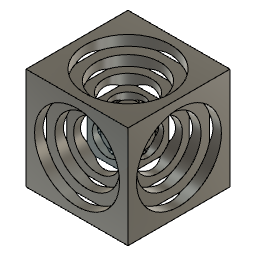
turnerscube (Autodesk Fusion 360 design; units mm, degrees)
Autodesk Fusion 360 part; units mm, degrees
note: some values were not read from the file. Set by a fixed rule: which sketch regions a step uses.
sketch "Sketch1" plane through (0, 0, 0) normal (0, 0, 1) x (1, 0, 0)
  line L0 (0, 0) -> (30, 0)
  line L1 (30, 0) -> (30, 30)
  line L2 (30, 30) -> (0, 30)
  line L3 (0, 30) -> (0, 0)
  dimension "d1" = 30
  dimension "d2" = 30
  constraint horizontal L0
  constraint vertical L1
  constraint horizontal L2
  constraint vertical L3
  constraint coincident L0.start L3.end
  measures "d1" distance of L0.start L2.end
  measures "d2" distance of L0.start L0.end
extrude "Extrude1" add sketch "Sketch1" along normal blind 30
sketch "Sketch2" plane through (30, 0, 0) normal (1, 0, 0) x (0, 1, 0)
  line L0 (0, 0) -> (30, 0)
  line L1 (30, 0) -> (30, 30)
  line L2 (30, 30) -> (0, 30)
  line L3 (0, 30) -> (0, 0)
  circle A0 centre (15, 15) radius 12.5
  line L4 (15, 30) -> (15, 0)
  dimension "d5" = 25
  constraint midpoint L2 L4.start
  constraint midpoint L0 L4.end
  constraint coincident A0.centre L4
  constraint midpoint A0.centre L4
  measures "d5" diameter of A0
  measures "d43" diameter of L2.end
sketch "Sketch3" plane through (0, 0, 30) normal (0, 0, 1) x (-1, 0, 0)
  line L0 (0, -30) -> (0, 0)
  line L1 (0, 0) -> (-30, 0)
  line L2 (-30, 0) -> (-30, -30)
  line L3 (-30, -30) -> (0, -30)
  circle A0 centre (-15, -15) radius 12.5
  line L4 (-15, -30) -> (-15, 0)
  dimension "d6" = 25
  constraint midpoint L3 L4.start
  constraint midpoint L1 L4.end
  constraint midpoint A0.centre L4
  measures "d6" diameter of A0
sketch "Sketch4" plane through (0, 0, 0) normal (0, -1, 0) x (1, 0, 0)
  line L0 (0, 0) -> (30, 0)
  line L1 (30, 0) -> (30, 30)
  line L2 (30, 30) -> (0, 30)
  line L3 (0, 30) -> (0, 0)
  circle A0 centre (15, 15) radius 12.5
  line L4 (15, 30) -> (15, 0)
  dimension "d7" = 25
  constraint midpoint L2 L4.start
  constraint midpoint L0 L4.end
  constraint midpoint A0.centre L4
  measures "d7" diameter of A0
sketch "Sketch5" plane through (0, 30, 0) normal (0, 1, 0) x (-1, 0, 0)
  line L0 (-30, 0) -> (0, 0)
  line L1 (0, 0) -> (0, 30)
  line L2 (0, 30) -> (-30, 30)
  line L3 (-30, 30) -> (-30, 0)
  circle A0 centre (-15, 15) radius 12.5
  line L4 (-15, 30) -> (-15, 0)
  dimension "d8" = 25
  constraint midpoint L2 L4.start
  constraint midpoint L0 L4.end
  constraint midpoint A0.centre L4
  measures "d8" diameter of A0
sketch "Sketch6" plane through (0, 0, 0) normal (-1, 0, 0) x (0, -1, 0)
  line L0 (-30, 0) -> (0, 0)
  line L1 (0, 0) -> (0, 30)
  line L2 (0, 30) -> (-30, 30)
  line L3 (-30, 30) -> (-30, 0)
  line L4 (-15, 30) -> (-15, 0)
  circle A0 centre (-15, 15) radius 12.5
  dimension "d9" = 25
  constraint midpoint L2 L4.start
  constraint midpoint L0 L4.end
  constraint midpoint L4 A0.centre
  measures "d9" diameter of A0
sketch "Sketch7" plane through (0, 0, 0) normal (0, 0, -1) x (1, 0, 0)
  line L0 (0, 0) -> (0, -30)
  line L1 (0, -30) -> (30, -30)
  line L2 (30, -30) -> (30, 0)
  line L3 (30, 0) -> (0, 0)
  line L4 (15, 0) -> (15, -30)
  circle A0 centre (15, -15) radius 12.5
  dimension "d10" = 25
  constraint midpoint L3 L4.start
  constraint midpoint L1 L4.end
  constraint midpoint L4 A0.centre
  measures "d10" diameter of A0
extrude "Extrude2" cut sketch "Sketch2" against normal blind 3 contours A0 L4 | A0 L4
extrude "Extrude3" cut sketch "Sketch4" against normal blind 3 contours A0 L4 | A0 L4
extrude "Extrude4" cut sketch "Sketch3" against normal blind 3 contours A0 L4 | A0 L4
extrude "Extrude5" cut sketch "Sketch5" against normal blind 3 contours A0 L4 | A0 L4
extrude "Extrude6" cut sketch "Sketch7" against normal blind 3 contours L4 A0 | L4 A0
extrude "Extrude7" cut sketch "Sketch6" against normal blind 3 contours L4 A0 | L4 A0
sketch "Sketch8" plane through (27, 0, 0) normal (1, 0, 0) x (0, 1, 0)
  line L0 (11.5, 3) -> (18.5, 3)
  arc A0 (18.5, 3) -> (27, 11.5) centre (15, 15) ccw
  line L1 (27, 11.5) -> (27, 18.5)
  arc A1 (27, 18.5) -> (18.5, 27) centre (15, 15) ccw
  line L2 (18.5, 27) -> (11.5, 27)
  arc A2 (11.5, 27) -> (3, 18.5) centre (15, 15) ccw
  line L3 (3, 18.5) -> (3, 11.5)
  arc A3 (3, 11.5) -> (11.5, 3) centre (15, 15) ccw
  circle A4 centre (15, 15) radius 9.5
  line L4 (15, 27) -> (15, 3)
  dimension "d23" = 19
  constraint midpoint L2 L4.start
  constraint midpoint L0 L4.end
  constraint midpoint A0.centre L4
  measures "d23" diameter of A4
sketch "Sketch9" plane through (0, 0, 27) normal (0, 0, 1) x (-1, 0, 0)
  line L0 (-3, -18.5) -> (-3, -11.5)
  arc A0 (-3, -11.5) -> (-11.5, -3) centre (-15, -15) ccw
  line L1 (-11.5, -3) -> (-18.5, -3)
  arc A1 (-18.5, -3) -> (-27, -11.5) centre (-15, -15) ccw
  line L2 (-27, -11.5) -> (-27, -18.5)
  arc A2 (-27, -18.5) -> (-18.5, -27) centre (-15, -15) ccw
  line L3 (-18.5, -27) -> (-11.5, -27)
  arc A3 (-11.5, -27) -> (-3, -18.5) centre (-15, -15) ccw
  line L4 (-15, -27) -> (-15, -3)
  circle A4 centre (-15, -15) radius 9.5
  dimension "d24" = 19
  constraint midpoint L3 L4.start
  constraint midpoint L1 L4.end
  constraint midpoint L4 A0.centre
  measures "d24" diameter of A4
sketch "Sketch10" plane through (0, 3, 0) normal (0, -1, 0) x (1, 0, 0)
  line L0 (3, 18.5) -> (3, 11.5)
  arc A0 (3, 11.5) -> (11.5, 3) centre (15, 15) ccw
  line L1 (11.5, 3) -> (18.5, 3)
  arc A1 (18.5, 3) -> (27, 11.5) centre (15, 15) ccw
  line L2 (27, 11.5) -> (27, 18.5)
  arc A2 (27, 18.5) -> (18.5, 27) centre (15, 15) ccw
  line L3 (18.5, 27) -> (11.5, 27)
  arc A3 (11.5, 27) -> (3, 18.5) centre (15, 15) ccw
  line L4 (15, 27) -> (15, 3)
  circle A4 centre (15, 15) radius 9.5
  dimension "d25" = 19
  constraint midpoint L3 L4.start
  constraint midpoint L1 L4.end
  constraint midpoint L4 A0.centre
  measures "d25" diameter of A4
sketch "Sketch11" plane through (3, 0, 0) normal (-1, 0, 0) x (0, -1, 0)
  line L0 (-18.5, 3) -> (-11.5, 3)
  arc A0 (-11.5, 3) -> (-3, 11.5) centre (-15, 15) ccw
  line L1 (-3, 11.5) -> (-3, 18.5)
  arc A1 (-3, 18.5) -> (-11.5, 27) centre (-15, 15) ccw
  line L2 (-11.5, 27) -> (-18.5, 27)
  arc A2 (-18.5, 27) -> (-27, 18.5) centre (-15, 15) ccw
  line L3 (-27, 18.5) -> (-27, 11.5)
  arc A3 (-27, 11.5) -> (-18.5, 3) centre (-15, 15) ccw
  line L4 (-15, 27) -> (-15, 3)
  circle A4 centre (-15, 15) radius 9.5
  dimension "d26" = 19
  constraint midpoint L2 L4.start
  constraint midpoint L0 L4.end
  constraint midpoint L4 A0.centre
  measures "d26" diameter of A4
sketch "Sketch12" plane through (0, 27, 0) normal (0, 1, 0) x (-1, 0, 0)
  line L0 (-3, 11.5) -> (-3, 18.5)
  arc A0 (-3, 18.5) -> (-11.5, 27) centre (-15, 15) ccw
  line L1 (-11.5, 27) -> (-18.5, 27)
  arc A1 (-18.5, 27) -> (-27, 18.5) centre (-15, 15) ccw
  line L2 (-27, 18.5) -> (-27, 11.5)
  arc A2 (-27, 11.5) -> (-18.5, 3) centre (-15, 15) ccw
  line L3 (-18.5, 3) -> (-11.5, 3)
  arc A3 (-11.5, 3) -> (-3, 11.5) centre (-15, 15) ccw
  line L4 (-15, 27) -> (-15, 3)
  circle A4 centre (-15, 15) radius 9.5
  dimension "d27" = 19
  constraint midpoint L1 L4.start
  constraint midpoint L3 L4.end
  constraint concentric A0 A4
  measures "d27" diameter of A4
sketch "Sketch13" plane through (0, 0, 3) normal (0, 0, -1) x (1, 0, 0)
  line L0 (3, -11.5) -> (3, -18.5)
  arc A0 (3, -18.5) -> (11.5, -27) centre (15, -15) ccw
  line L1 (11.5, -27) -> (18.5, -27)
  arc A1 (18.5, -27) -> (27, -18.5) centre (15, -15) ccw
  line L2 (27, -18.5) -> (27, -11.5)
  arc A2 (27, -11.5) -> (18.5, -3) centre (15, -15) ccw
  line L3 (18.5, -3) -> (11.5, -3)
  arc A3 (11.5, -3) -> (3, -11.5) centre (15, -15) ccw
  line L4 (15, -3) -> (15, -27)
  circle A4 centre (15, -15) radius 9.5
  dimension "d28" = 19
  constraint midpoint L3 L4.start
  constraint midpoint L1 L4.end
  constraint concentric A0 A4
  measures "d28" diameter of A4
extrude "Extrude8" cut sketch "Sketch13" against normal blind 3 contours L4 A4 | L4 A4
extrude "Extrude9" cut sketch "Sketch12" against normal blind 3 contours L4 A4 | L4 A4
extrude "Extrude10" cut sketch "Sketch9" against normal blind 3 contours L4 A4 | L4 A4
extrude "Extrude11" cut sketch "Sketch8" against normal blind 3 contours A4 L4 | A4 L4
extrude "Extrude12" cut sketch "Sketch10" against normal blind 3 contours L4 A4 | L4 A4
extrude "Extrude13" cut sketch "Sketch11" against normal blind 3 contours L4 A4 | L4 A4
sketch "Sketch14" plane through (0, 24, 0) normal (0, 1, 0) x (-1, 0, 0)
  line L0 (-6, 11.9586) -> (-6, 18.0414)
  arc A0 (-6, 18.0414) -> (-11.9586, 24) centre (-15, 15) ccw
  line L1 (-11.9586, 24) -> (-18.0414, 24)
  arc A1 (-18.0414, 24) -> (-24, 18.0414) centre (-15, 15) ccw
  line L2 (-24, 18.0414) -> (-24, 11.9586)
  arc A2 (-24, 11.9586) -> (-18.0414, 6) centre (-15, 15) ccw
  line L3 (-18.0414, 6) -> (-11.9586, 6)
  arc A3 (-11.9586, 6) -> (-6, 11.9586) centre (-15, 15) ccw
  line L4 (-15, 24) -> (-15, 6)
  circle A4 centre (-15, 15) radius 7
  dimension "d41" = 14
  constraint midpoint L1 L4.start
  constraint midpoint L3 L4.end
  constraint concentric A0 A4
  measures "d41" diameter of A4
sketch "Sketch15" plane through (6, 0, 0) normal (-1, 0, 0) x (0, -1, 0)
  line L0 (-6, 11.9586) -> (-6, 18.0414)
  arc A0 (-6, 18.0414) -> (-11.9586, 24) centre (-15, 15) ccw
  line L1 (-11.9586, 24) -> (-18.0414, 24)
  arc A1 (-18.0414, 24) -> (-24, 18.0414) centre (-15, 15) ccw
  line L2 (-24, 18.0414) -> (-24, 11.9586)
  arc A2 (-24, 11.9586) -> (-18.0414, 6) centre (-15, 15) ccw
  line L3 (-18.0414, 6) -> (-11.9586, 6)
  arc A3 (-11.9586, 6) -> (-6, 11.9586) centre (-15, 15) ccw
  line L4 (-15, 24) -> (-15, 6)
  circle A4 centre (-15, 15) radius 7
  dimension "d42" = 14
  constraint midpoint L1 L4.start
  constraint midpoint L3 L4.end
  constraint concentric A0 A4
  measures "d42" diameter of A4
sketch "Sketch16" plane through (0, 6, 0) normal (0, -1, 0) x (1, 0, 0)
  line L0 (6, 18.0414) -> (6, 11.9586)
  arc A0 (6, 11.9586) -> (11.9586, 6) centre (15, 15) ccw
  line L1 (11.9586, 6) -> (18.0414, 6)
  arc A1 (18.0414, 6) -> (24, 11.9586) centre (15, 15) ccw
  line L2 (24, 11.9586) -> (24, 18.0414)
  arc A2 (24, 18.0414) -> (18.0414, 24) centre (15, 15) ccw
  line L3 (18.0414, 24) -> (11.9586, 24)
  arc A3 (11.9586, 24) -> (6, 18.0414) centre (15, 15) ccw
  line L4 (15, 24) -> (15, 6)
  circle A4 centre (15, 15) radius 7
  dimension "d43" = 14
  constraint midpoint L3 L4.start
  constraint midpoint L1 L4.end
  constraint concentric A0 A4
  measures "d43" diameter of A4
sketch "Sketch17" plane through (24, 0, 0) normal (1, 0, 0) x (0, 1, 0)
  line L0 (6, 18.0414) -> (6, 11.9586)
  arc A0 (6, 11.9586) -> (11.9586, 6) centre (15, 15) ccw
  line L1 (11.9586, 6) -> (18.0414, 6)
  arc A1 (18.0414, 6) -> (24, 11.9586) centre (15, 15) ccw
  line L2 (24, 11.9586) -> (24, 18.0414)
  arc A2 (24, 18.0414) -> (18.0414, 24) centre (15, 15) ccw
  line L3 (18.0414, 24) -> (11.9586, 24)
  arc A3 (11.9586, 24) -> (6, 18.0414) centre (15, 15) ccw
  line L4 (15, 24) -> (15, 6)
  circle A4 centre (15, 15) radius 7
  dimension "d44" = 14
  constraint midpoint L3 L4.start
  constraint midpoint L1 L4.end
  constraint concentric A0 A4
  measures "d44" diameter of A4
sketch "Sketch18" plane through (0, 0, 24) normal (0, 0, 1) x (-1, 0, 0)
  line L0 (-6, -18.0414) -> (-6, -11.9586)
  arc A0 (-6, -11.9586) -> (-11.9586, -6) centre (-15, -15) ccw
  line L1 (-11.9586, -6) -> (-18.0414, -6)
  arc A1 (-18.0414, -6) -> (-24, -11.9586) centre (-15, -15) ccw
  line L2 (-24, -11.9586) -> (-24, -18.0414)
  arc A2 (-24, -18.0414) -> (-18.0414, -24) centre (-15, -15) ccw
  line L3 (-18.0414, -24) -> (-11.9586, -24)
  arc A3 (-11.9586, -24) -> (-6, -18.0414) centre (-15, -15) ccw
  line L4 (-15, -24) -> (-15, -6)
  circle A4 centre (-15, -15) radius 7
  dimension "d45" = 14
  constraint midpoint L3 L4.start
  constraint midpoint L1 L4.end
  constraint concentric A0 A4
  measures "d45" diameter of A4
sketch "Sketch19" plane through (0, 0, 6) normal (0, 0, -1) x (1, 0, 0)
  line L0 (6, -11.9586) -> (6, -18.0414)
  arc A0 (6, -18.0414) -> (11.9586, -24) centre (15, -15) ccw
  line L1 (11.9586, -24) -> (18.0414, -24)
  arc A1 (18.0414, -24) -> (24, -18.0414) centre (15, -15) ccw
  line L2 (24, -18.0414) -> (24, -11.9586)
  arc A2 (24, -11.9586) -> (18.0414, -6) centre (15, -15) ccw
  line L3 (18.0414, -6) -> (11.9586, -6)
  arc A3 (11.9586, -6) -> (6, -11.9586) centre (15, -15) ccw
  line L4 (15, -6) -> (15, -24)
  circle A4 centre (15, -15) radius 7
  dimension "d46" = 14
  constraint midpoint L3 L4.start
  constraint midpoint L1 L4.end
  constraint concentric A0 A4
  measures "d46" diameter of A4
extrude "Extrude14" cut sketch "Sketch18" against normal blind 3 contours L4 A4 | L4 A4
extrude "Extrude15" cut sketch "Sketch17" against normal blind 3 contours L4 A4 | L4 A4
extrude "Extrude16" cut sketch "Sketch16" against normal blind 3 contours L4 A4 | L4 A4
extrude "Extrude17" cut sketch "Sketch15" against normal blind 3 contours L4 A4 | L4 A4
extrude "Extrude18" cut sketch "Sketch14" against normal blind 3 contours L4 A4 | L4 A4
extrude "Extrude19" cut sketch "Sketch19" against normal blind 3 contours L4 A4 | L4 A4
sketch "Sketch20" plane through (0, 9, 0) normal (0, -1, 0) x (1, 0, 0)
  line L0 (11.3944, 9) -> (18.6056, 9)
  arc A0 (18.6056, 9) -> (21, 11.3944) centre (15, 15) ccw
  line L1 (21, 11.3944) -> (21, 18.6056)
  arc A1 (21, 18.6056) -> (18.6056, 21) centre (15, 15) ccw
  line L2 (18.6056, 21) -> (11.3944, 21)
  arc A2 (11.3944, 21) -> (9, 18.6056) centre (15, 15) ccw
  line L3 (9, 18.6056) -> (9, 11.3944)
  arc A3 (9, 11.3944) -> (11.3944, 9) centre (15, 15) ccw
sketch "Sketch21" plane through (0, 9, 0) normal (0, -1, 0) x (1, 0, 0)
  line L0 (15, 21) -> (15, 9)
  circle A0 centre (15, 15) radius 4.5
  dimension "d59" = 9
  constraint vertical L0
  constraint midpoint L0 A0.centre
  measures "d59" diameter of A0
sketch "Sketch22" plane through (21, 0, 0) normal (1, 0, 0) x (0, 1, 0)
  line L0 (11.3944, 9) -> (18.6056, 9)
  arc A0 (18.6056, 9) -> (21, 11.3944) centre (15, 15) ccw
  line L1 (21, 11.3944) -> (21, 18.6056)
  arc A1 (21, 18.6056) -> (18.6056, 21) centre (15, 15) ccw
  line L2 (18.6056, 21) -> (11.3944, 21)
  arc A2 (11.3944, 21) -> (9, 18.6056) centre (15, 15) ccw
  line L3 (9, 18.6056) -> (9, 11.3944)
  arc A3 (9, 11.3944) -> (11.3944, 9) centre (15, 15) ccw
  line L4 (15, 21) -> (15, 9)
  circle A4 centre (15, 15) radius 4.5
  dimension "d60" = 9
  constraint midpoint L2 L4.start
  constraint midpoint L0 L4.end
  constraint concentric A0 A4
  measures "d60" diameter of A4
sketch "Sketch23" plane through (0, 21, 0) normal (0, 1, 0) x (-1, 0, 0)
  line L0 (-18.6056, 9) -> (-11.3944, 9)
  arc A0 (-11.3944, 9) -> (-9, 11.3944) centre (-15, 15) ccw
  line L1 (-9, 11.3944) -> (-9, 18.6056)
  arc A1 (-9, 18.6056) -> (-11.3944, 21) centre (-15, 15) ccw
  line L2 (-11.3944, 21) -> (-18.6056, 21)
  arc A2 (-18.6056, 21) -> (-21, 18.6056) centre (-15, 15) ccw
  line L3 (-21, 18.6056) -> (-21, 11.3944)
  arc A3 (-21, 11.3944) -> (-18.6056, 9) centre (-15, 15) ccw
  line L4 (-15, 21) -> (-15, 9)
  circle A4 centre (-15, 15) radius 4.5
  dimension "d61" = 9
  constraint midpoint L2 L4.start
  constraint midpoint L0 L4.end
  constraint concentric A0 A4
  measures "d61" diameter of A4
sketch "Sketch24" plane through (9, 0, 0) normal (-1, 0, 0) x (0, -1, 0)
  line L0 (-18.6056, 9) -> (-11.3944, 9)
  arc A0 (-11.3944, 9) -> (-9, 11.3944) centre (-15, 15) ccw
  line L1 (-9, 11.3944) -> (-9, 18.6056)
  arc A1 (-9, 18.6056) -> (-11.3944, 21) centre (-15, 15) ccw
  line L2 (-11.3944, 21) -> (-18.6056, 21)
  arc A2 (-18.6056, 21) -> (-21, 18.6056) centre (-15, 15) ccw
  line L3 (-21, 18.6056) -> (-21, 11.3944)
  arc A3 (-21, 11.3944) -> (-18.6056, 9) centre (-15, 15) ccw
  line L4 (-15, 21) -> (-15, 9)
  circle A4 centre (-15, 15) radius 4.5
  dimension "d62" = 9
  constraint midpoint L2 L4.start
  constraint midpoint L0 L4.end
  constraint concentric A0 A4
  measures "d62" diameter of A4
sketch "Sketch25" plane through (0, 0, 21) normal (0, 0, 1) x (-1, 0, 0)
  line L0 (-18.6056, -21) -> (-11.3944, -21)
  arc A0 (-11.3944, -21) -> (-9, -18.6056) centre (-15, -15) ccw
  line L1 (-9, -18.6056) -> (-9, -11.3944)
  arc A1 (-9, -11.3944) -> (-11.3944, -9) centre (-15, -15) ccw
  line L2 (-11.3944, -9) -> (-18.6056, -9)
  arc A2 (-18.6056, -9) -> (-21, -11.3944) centre (-15, -15) ccw
  line L3 (-21, -11.3944) -> (-21, -18.6056)
  arc A3 (-21, -18.6056) -> (-18.6056, -21) centre (-15, -15) ccw
  line L4 (-15, -21) -> (-15, -9)
  circle A4 centre (-15, -15) radius 4.5
  dimension "d63" = 9
  constraint midpoint L0 L4.start
  constraint midpoint L2 L4.end
  constraint concentric A0 A4
  measures "d63" diameter of A4
sketch "Sketch26" plane through (0, 0, 9) normal (0, 0, -1) x (1, 0, 0)
  line L0 (11.3944, -21) -> (18.6056, -21)
  arc A0 (18.6056, -21) -> (21, -18.6056) centre (15, -15) ccw
  line L1 (21, -18.6056) -> (21, -11.3944)
  arc A1 (21, -11.3944) -> (18.6056, -9) centre (15, -15) ccw
  line L2 (18.6056, -9) -> (11.3944, -9)
  arc A2 (11.3944, -9) -> (9, -11.3944) centre (15, -15) ccw
  line L3 (9, -11.3944) -> (9, -18.6056)
  arc A3 (9, -18.6056) -> (11.3944, -21) centre (15, -15) ccw
  line L4 (15, -9) -> (15, -21)
  circle A4 centre (15, -15) radius 4.5
  dimension "d64" = 9
  constraint midpoint L2 L4.start
  constraint midpoint L0 L4.end
  constraint concentric A0 A4
  measures "d64" diameter of A4
extrude "Extrude20" cut sketch "Sketch24" against normal blind 2 contours L4 A4 | L4 A4
extrude "Extrude21" cut sketch "Sketch21" against normal blind 2
extrude "Extrude22" cut sketch "Sketch22" against normal blind 2 contours L4 A4 | L4 A4
extrude "Extrude23" cut sketch "Sketch23" against normal blind 2 contours L4 A4 | L4 A4
extrude "Extrude24" cut sketch "Sketch25" against normal blind 2 contours L4 A4 | L4 A4
extrude "Extrude25" cut sketch "Sketch26" against normal blind 2 contours L4 A4 | L4 A4
sketch "Sketch27" plane through (19, 0, 0) normal (1, 0, 0) x (0, 1, 0)
  line L0 (12.9384, 11) -> (17.0616, 11)
  arc A0 (17.0616, 11) -> (19, 12.9384) centre (15, 15) ccw
  line L1 (19, 12.9384) -> (19, 17.0616)
  arc A1 (19, 17.0616) -> (17.0616, 19) centre (15, 15) ccw
  line L2 (17.0616, 19) -> (12.9384, 19)
  arc A2 (12.9384, 19) -> (11, 17.0616) centre (15, 15) ccw
  line L3 (11, 17.0616) -> (11, 12.9384)
  arc A3 (11, 12.9384) -> (12.9384, 11) centre (15, 15) ccw
  line L4 (15, 19) -> (15, 11)
  circle A4 centre (15, 15) radius 2.5
  dimension "d77" = 5
  constraint midpoint L2 L4.start
  constraint midpoint L0 L4.end
  constraint concentric A0 A4
  measures "d77" diameter of A4
sketch "Sketch28" plane through (0, 19, 0) normal (0, 1, 0) x (-1, 0, 0)
  line L0 (-17.0616, 11) -> (-12.9384, 11)
  arc A0 (-12.9384, 11) -> (-11, 12.9384) centre (-15, 15) ccw
  line L1 (-11, 12.9384) -> (-11, 17.0616)
  arc A1 (-11, 17.0616) -> (-12.9384, 19) centre (-15, 15) ccw
  line L2 (-12.9384, 19) -> (-17.0616, 19)
  arc A2 (-17.0616, 19) -> (-19, 17.0616) centre (-15, 15) ccw
  line L3 (-19, 17.0616) -> (-19, 12.9384)
  arc A3 (-19, 12.9384) -> (-17.0616, 11) centre (-15, 15) ccw
  line L4 (-15, 19) -> (-15, 11)
  circle A4 centre (-15, 15) radius 2.5
  dimension "d78" = 5
  constraint midpoint L2 L4.start
  constraint midpoint L0 L4.end
  constraint concentric A0 A4
  measures "d78" diameter of A4
sketch "Sketch29" plane through (11, 0, 0) normal (-1, 0, 0) x (0, -1, 0)
  line L0 (-17.0616, 11) -> (-12.9384, 11)
  arc A0 (-12.9384, 11) -> (-11, 12.9384) centre (-15, 15) ccw
  line L1 (-11, 12.9384) -> (-11, 17.0616)
  arc A1 (-11, 17.0616) -> (-12.9384, 19) centre (-15, 15) ccw
  line L2 (-12.9384, 19) -> (-17.0616, 19)
  arc A2 (-17.0616, 19) -> (-19, 17.0616) centre (-15, 15) ccw
  line L3 (-19, 17.0616) -> (-19, 12.9384)
  arc A3 (-19, 12.9384) -> (-17.0616, 11) centre (-15, 15) ccw
  line L4 (-15, 19) -> (-15, 11)
  circle A4 centre (-15, 15) radius 2.5
  dimension "d79" = 5
  constraint midpoint L2 L4.start
  constraint midpoint L0 L4.end
  constraint concentric A0 A4
  measures "d79" diameter of A4
sketch "Sketch30" plane through (0, 0, 19) normal (0, 0, 1) x (-1, 0, 0)
  line L0 (-17.0616, -19) -> (-12.9384, -19)
  arc A0 (-12.9384, -19) -> (-11, -17.0616) centre (-15, -15) ccw
  line L1 (-11, -17.0616) -> (-11, -12.9384)
  arc A1 (-11, -12.9384) -> (-12.9384, -11) centre (-15, -15) ccw
  line L2 (-12.9384, -11) -> (-17.0616, -11)
  arc A2 (-17.0616, -11) -> (-19, -12.9384) centre (-15, -15) ccw
  line L3 (-19, -12.9384) -> (-19, -17.0616)
  arc A3 (-19, -17.0616) -> (-17.0616, -19) centre (-15, -15) ccw
  line L4 (-15, -19) -> (-15, -11)
  circle A4 centre (-15, -15) radius 2.5
  dimension "d80" = 5
  constraint midpoint L0 L4.start
  constraint midpoint L2 L4.end
  constraint concentric A0 A4
  measures "d80" diameter of A4
sketch "Sketch31" plane through (0, 0, 11) normal (0, 0, -1) x (1, 0, 0)
  line L0 (12.9384, -19) -> (17.0616, -19)
  arc A0 (17.0616, -19) -> (19, -17.0616) centre (15, -15) ccw
  line L1 (19, -17.0616) -> (19, -12.9384)
  arc A1 (19, -12.9384) -> (17.0616, -11) centre (15, -15) ccw
  line L2 (17.0616, -11) -> (12.9384, -11)
  arc A2 (12.9384, -11) -> (11, -12.9384) centre (15, -15) ccw
  line L3 (11, -12.9384) -> (11, -17.0616)
  arc A3 (11, -17.0616) -> (12.9384, -19) centre (15, -15) ccw
  line L4 (15, -11) -> (15, -19)
  circle A4 centre (15, -15) radius 2.5
  dimension "d81" = 5
  constraint midpoint L2 L4.start
  constraint midpoint L0 L4.end
  constraint concentric A0 A4
  measures "d81" diameter of A4
extrude "Extrude26" cut sketch "Sketch27" against normal blind 3 contours L4 A4 | L4 A4
extrude "Extrude27" cut sketch "Sketch28" against normal blind 3 contours L4 A4 | L4 A4
extrude "Extrude28" cut sketch "Sketch29" against normal blind 3 contours L4 A4 | L4 A4
extrude "Extrude29" cut sketch "Sketch30" against normal blind 3 contours L4 A4 | L4 A4
extrude "Extrude30" cut sketch "Sketch31" against normal blind 3 contours L4 A4 | L4 A4
sketch "Sketch32" plane through (15, 9, 15) normal (0, -1, 0) x (1, 0, 0)
  line L0 (0, 4) -> (0, -4)
  circle A0 centre (0, 0) radius 2.5
  dimension "d92" = 5
  constraint vertical L0
  constraint coincident A0.centre origin
  measures "d92" diameter of A0
extrude "Extrude31" cut sketch "Sketch32" against normal blind 10
